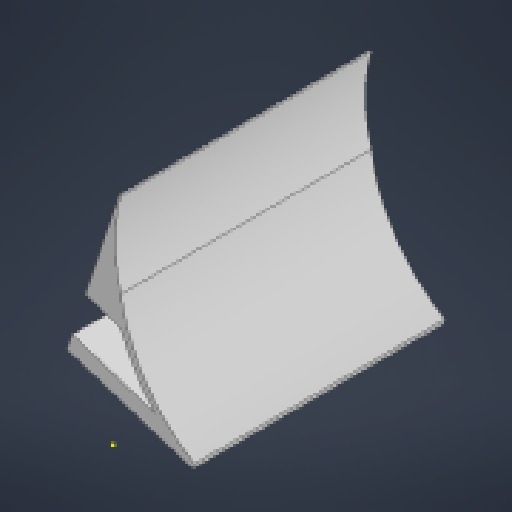
# Autodesk Inventor part: загиб 20-25
Saved by Autodesk Inventor 2025 (Build 290162000, 162)
## iProperties
Created: 2025-10-03
Part Number: загиб 20-25
Material: Типовые
Document SubType Name: Modeling
Designer: Phantom
Density: 1 g/cm^3
Appearance: По умолчанию
Author: Phantom
Autodesk Inventor part; units mm, degrees
ref_plane "YZ Plane" through (0, 0, 0) normal (1, 0, 0) x (0, 1, 0)
ref_plane "XZ Plane" through (0, 0, 0) normal (0, 1, 0) x (-1, 0, 0)
ref_plane "XY Plane" through (0, 0, 0) normal (0, 0, 1) x (1, 0, 0)
sketch "Эскиз1" plane through (0, 0, 0) normal (0, 0, 1) x (1, 0, 0)
  line L0 (14.551272, 220.323529) -> (16.668611, 220.303571)
  line L1 (220, 0) -> (230, 0) construction
  line L2 (0, 0) -> (170, 0)
  line L3 (170, 0) -> (170, 2)
  arc A0 (14.551272, 220.323529) -> (170, 0) centre (170, 165) ccw
  arc A1 (16.668611, 220.303571) -> (170, 2) centre (170, 165) ccw
  line L4 (170, 1) -> (170, 0)
  dimension "d12" = 330
  dimension "d13" = 2
  constraints: 10 end point, 4 point on circle, 2 centre point, 2 horizontal, 1 midpoint, 1 vertical
  measures "d12" diameter of A0
  measures "d13" radial gap between concentric circles of A0 A1
extrude "Выдавливание1" add sketch "Эскиз1" along normal blind 385
sketch "Эскиз2" plane through (0, 0, 0) normal (0, 0, -1) x (-1, 0, 0)
  line L0 (-16.668611, 220.303571) -> (-14.551272, 220.323529)
  arc A0 (-170, 2) -> (-16.668611, 220.303571) centre (-170, 165) ccw
  line L1 (-170, 0) -> (-170, 2)
  arc A1 (-170, 0) -> (-14.551272, 220.323529) centre (-170, 165) ccw
  point P0 (0, 0)
extrude "Выдавливание2" cut sketch "Эскиз2" against normal blind 121
chamfer "Фаска1" distance 2 angle 45 1 edges at (170, 2, 253)
chamfer "Фаска2" distance 2.8 angle 45 1 edges at (168.0001, 2.0123, 253)
sketch "Эскиз4" plane through (0, 0, 385) normal (0, 0, 1) x (1, 0, 0)
  line L0 (165.200647, 2.070671) -> (169.973854, 0.026307)
  arc A0 (16.668611, 220.303571) -> (165.200647, 2.070671) centre (170, 165) ccw
  line L1 (16.668611, 220.303571) -> (14.551272, 220.323529)
  arc A1 (14.551272, 220.323529) -> (170, 0) centre (170, 165) ccw
  line L2 (169.973854, 0.026307) -> (170, 0)
  arc A2 (8.479952, 230.770296) -> (172.192867, 23.682282) centre (165.36401, 186.539172) ccw
  arc A3 (6.366578, 230.639248) -> (177.127636, 21.959048) centre (165.36401, 186.539172) ccw
  line L3 (8.479952, 230.770296) -> (6.366578, 230.639248)
  point P0 (0, 0)
  point P1 (6.735972, 141.128316)
  point P2 (5.243718, 156.035199)
extrude "Выдавливание3" add sketch "Эскиз4" against normal up to surface (264 mm away) contours A3 L3 A2 A1
sketch "Эскиз5" plane through (0, 0, 385) normal (0, 0, 1) x (1, 0, 0)
  point P0 (0, 0)
sketch "Эскиз6" plane through (0, 0, 385) normal (0, 0, 1) x (1, 0, 0)
  arc A0 (8.479952, 230.770296) -> (172.192867, 23.682282) centre (165.36401, 186.539172) ccw
  arc A1 (4.217365, 151.088374) -> (177.127636, 21.959048) centre (165.36401, 186.539172) ccw
  arc A2 (6.366578, 230.639248) -> (6.735972, 141.128316) centre (165.36401, 186.539172) ccw
  line L0 (8.479952, 230.770296) -> (6.366578, 230.639248)
  line L1 (165.200647, 2.070671) -> (169.973854, 0.026307)
  arc A3 (16.668611, 220.303571) -> (165.200647, 2.070671) centre (170, 165) ccw
  line L2 (16.668611, 220.303571) -> (14.551272, 220.323529)
  arc A4 (14.551272, 220.323529) -> (5.243718, 156.035199) centre (170, 165) ccw
  arc A5 (8.479952, 230.770296) -> (5.243718, 156.035199) centre (165.36401, 186.539172) ccw
  line L3 (8.479952, 230.770296) -> (6.366578, 230.639248)
  arc A6 (6.366578, 230.639248) -> (6.735972, 141.128316) centre (165.36401, 186.539172) ccw
  arc A7 (6.735972, 141.128316) -> (170, 0) centre (170, 165) ccw
  line L4 (169.973854, 0.026307) -> (170, 0)
  point P0 (0, 0)
  point P1 (5.243718, 156.035199)
  point P2 (8.695622, 141.550102)
extrude "Выдавливание4" cut sketch "Эскиз6" against normal through all contours A4 L2 A3 A0
sketch "Эскиз7" plane through (0, 0, 385) normal (0, 0, 1) x (1, 0, 0)
  arc A0 (8.479952, 230.770296) -> (8.695622, 141.550102) centre (165.36401, 186.539172) ccw
  line L0 (8.479952, 230.770296) -> (6.366578, 230.639248)
  arc A1 (6.366578, 230.639248) -> (6.735972, 141.128316) centre (165.36401, 186.539172) ccw
  arc A2 (6.735972, 141.128316) -> (170, 0) centre (170, 165) ccw
  line L1 (169.973854, 0.026307) -> (170, 0)
  line L2 (165.200647, 2.070671) -> (169.973854, 0.026307)
  arc A3 (8.695622, 141.550102) -> (165.200647, 2.070671) centre (170, 165) ccw
  line L3 (7.950702, 133.935149) -> (-40.099318, 149.531591)
  line L4 (-49.858035, 62.780108) -> (67.459858, 424.216841)
  line L5 (-49.858035, 62.780108) -> (127.054407, 5.686862)
  line L6 (-49.858035, 62.780108) -> (-48.005647, 68.487004)
  line L7 (-48.005647, 68.487004) -> (101.321571, 20.296071)
  line L8 (86.253826, 25.158739) -> (84.411089, 19.448728)
  line L9 (-13.720493, 69.363932) -> (64.107759, 44.247171)
  line L10 (-13.720493, 69.363932) -> (-53.207333, 82.107139)
  line L11 (6.366578, 230.639248) -> (-61.821222, 20.564085)
  line L12 (0.365434, 112.76031) -> (33.03639, 102.155722)
  line L13 (0.365434, 112.76031) -> (-39.196629, 125.601667)
  point P0 (0, 0)
  point P1 (-42.922459, 78.788001)
  point P2 (-48.283371, 62.271932)
  point P3 (85.623551, 23.205731)
  point P4 (54.225117, 47.4365)
  point P5 (-21.879547, 143.617679)
  point P6 (-28.820519, 122.23371)
  point P7 (15.175388, 107.953182)
  dimension "d24" = 6
  constraints: 20 end point, 4 parallel, 3 point on circle, 3 point on line, 2 perpendicular, 1 collinear, 2 other
  measures "d24" distance of L4.start L6.end
extrude "Выдавливание5" add sketch "Эскиз7" against normal up to surface (264 mm away) contours A1 A2 L3 L11 | L3 A2 L12 L13 L11 | A2 L7 L11 L10 L9 | A2 L8 L5 L11 L7
sketch "Эскиз8" plane through (0, 0, 385) normal (0, 0, 1) x (1, 0, 0)
  arc A0 (-12.527916, 69.511986) -> (1.243719, 111.94008) centre (-8.463622, 91.641865) ccw
  arc A1 (15.175388, 107.953182) -> (54.225117, 47.4365) centre (170, 165) ccw
  arc A2 (9.177094, 109.900154) -> (50.716787, 43.87397) centre (170, 165) ccw
  line L0 (-28.820519, 122.23371) -> (15.175388, 107.953182)
  line L1 (54.225117, 47.4365) -> (-42.922459, 78.788001)
  point P0 (0, 0)
  point P1 (44.18074, 50.678025)
  dimension "d27" = 5
  constraints: 2 point on circle, 1 centre point, 1 point on line
  measures "d27" radial gap between concentric circles of A1 A2
extrude "Выдавливание6" add sketch "Эскиз8" against normal up to surface (264 mm away)
sketch "Эскиз9" plane through (0, 0, 385) normal (0, 0, 1) x (1, 0, 0)
  arc A0 (8.479952, 230.770296) -> (8.695622, 141.550102) centre (165.36401, 186.539172) ccw
  line L0 (8.479952, 230.770296) -> (6.366578, 230.639248)
  line L1 (6.366578, 230.639248) -> (-28.820519, 122.23371)
  line L2 (-28.820519, 122.23371) -> (9.177094, 109.900154)
  arc A1 (9.177094, 109.900154) -> (44.18074, 50.678025) centre (170, 165) ccw
  line L3 (44.18074, 50.678025) -> (-42.922459, 78.788001)
  line L4 (-42.922459, 78.788001) -> (-48.283371, 62.271932)
  line L5 (-48.283371, 62.271932) -> (84.411089, 19.448728)
  line L6 (84.411089, 19.448728) -> (85.623551, 23.205731)
  arc A2 (85.623551, 23.205731) -> (170, 0) centre (170, 165) ccw
  line L7 (169.973854, 0.026307) -> (170, 0)
  line L8 (165.200647, 2.070671) -> (169.973854, 0.026307)
  arc A3 (8.695622, 141.550102) -> (165.200647, 2.070671) centre (170, 165) ccw
  line L9 (85.623551, 23.205731) -> (90.450352, 38.162337)
  line L10 (84.411089, 19.448728) -> (85.623551, 23.205731)
  point P0 (0, 0)
  point P1 (86.253826, 25.158739)
  constraints: 2 end point, 1 collinear
extrude "Выдавливание7" cut sketch "Эскиз9" against normal through all contours A3 L8 L7 A2 L9
